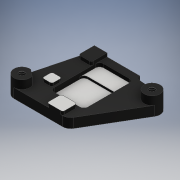
# Autodesk Inventor part: EPS_RegulatorHeatsink-A
Saved by Autodesk Inventor 2018 (Build 220112000, 112)
## iProperties
Created: 2018-09-29
Part Number: EPS_RegulatorHeatsink-A
Material: Aluminum 6061
Document SubType Name: Modeling
Designer: Bradley
Density: 2.7 g/cm^3
Appearance: Anodized - Dark Gray
Author: Bradley
Autodesk Inventor part; units mm, degrees
ref_plane "YZ Plane" through (0, 0, 0) normal (1, 0, 0) x (0, 1, 0)
ref_plane "XZ Plane" through (0, 0, 0) normal (0, 1, 0) x (-1, 0, 0)
ref_plane "XY Plane" through (0, 0, 0) normal (0, 0, 1) x (1, 0, 0)
sketch "Sketch9" plane through (0, 0, 0) normal (0, 0, 1) x (1, 0, 0)
  circle A0 centre (-9.3, -6.3) radius 2
  circle A1 centre (10.6, 6.6) radius 2
  line L0 (3.75, -3.75) -> (-3.75, -3.75) construction
  line L1 (-3.75, -3.75) -> (-3.75, 3.75) construction
  line L2 (-3.75, 3.75) -> (3.75, 3.75) construction
  line L3 (3.75, 3.75) -> (3.75, -3.75) construction
  line L4 (3.75, -3.75) -> (-3.75, 3.75) construction
  line L5 (-3.75, -3.75) -> (3.75, 3.75) construction
  line L6 (-4.95, -3.125) -> (-6.85, -3.125) construction
  line L7 (-6.85, -3.125) -> (-6.85, -1.175) construction
  line L8 (-6.85, -1.175) -> (-4.95, -1.175) construction
  line L9 (-4.95, -1.175) -> (-4.95, -3.125) construction
  line L10 (-4.95, -3.125) -> (-6.85, -1.175) construction
  line L11 (-6.85, -3.125) -> (-4.95, -1.175) construction
  line L12 (2.575, -4.925) -> (-0.575, -4.925) construction
  line L13 (-0.575, -4.925) -> (-0.575, -8.075) construction
  line L14 (-0.575, -8.075) -> (2.575, -8.075) construction
  line L15 (2.575, -8.075) -> (2.575, -4.925) construction
  line L16 (2.575, -4.925) -> (-0.575, -8.075) construction
  line L17 (-0.575, -4.925) -> (2.575, -8.075) construction
  line L18 (12.3232, 5.5848) -> (4.7232, -7.3152)
  arc A2 (3, -8.3) -> (4.7232, -7.3152) centre (3, -6.3) ccw
  line L19 (3, -8.3) -> (-9.3, -8.3)
  line L20 (-11.2363, -5.7994) -> (-7.5137, 8.5994)
  arc A3 (-7.5137, 8.5994) -> (-7.45, 9.1) centre (-9.45, 9.1) ccw
  line L21 (-7.45, 9.1) -> (-7.45, 10.1)
  line L22 (-7.45, 10.1) -> (4, 10.1)
  arc A4 (4, 10.1) -> (4.9131, 9.1038) centre (5, 10.1) ccw
  line L23 (4.9131, 9.1038) -> (10.7738, 8.5924)
  line L24 (3.25, -4.25) -> (-3.25, -4.25)
  line L25 (-4.25, -3.25) -> (-4.25, 3.25)
  line L26 (-3.25, 4.25) -> (3.25, 4.25)
  line L27 (4.25, 3.25) -> (4.25, -3.25)
  arc A5 (3.25, -4.25) -> (4.25, -3.25) centre (3.25, -3.25) ccw
  arc A6 (-4.25, -3.25) -> (-3.25, -4.25) centre (-3.25, -3.25) ccw
  arc A7 (-3.25, 4.25) -> (-4.25, 3.25) centre (-3.25, 3.25) ccw
  arc A8 (4.25, 3.25) -> (3.25, 4.25) centre (3.25, 3.25) ccw
  line L28 (1.7, 7.8) -> (-2.3, 7.8) construction
  line L29 (-2.3, 7.8) -> (-2.3, 5) construction
  line L30 (-2.3, 5) -> (1.7, 5) construction
  line L31 (1.7, 5) -> (1.7, 7.8) construction
  line L32 (1.7, 7.8) -> (-2.3, 5) construction
  line L33 (-2.3, 7.8) -> (1.7, 5) construction
  line L34 (-4.25, 3.25) -> (-4.25, 7.2)
  arc A9 (-3.25, 8.2) -> (-4.25, 7.2) centre (-3.25, 7.2) ccw
  line L35 (-3.25, 8.2) -> (3.25, 8.2)
  arc A10 (4.25, 7.2) -> (3.25, 8.2) centre (3.25, 7.2) ccw
  line L36 (4.25, 7.2) -> (4.25, 3.25)
  line L37 (-5.15, -3.4) -> (-6.65, -3.4)
  line L38 (-7.15, -2.9) -> (-7.15, -1.4)
  line L39 (-6.65, -0.9) -> (-5.15, -0.9)
  line L40 (-4.65, -1.4) -> (-4.65, -2.9)
  arc A11 (-5.15, -3.4) -> (-4.65, -2.9) centre (-5.15, -2.9) ccw
  arc A12 (-4.65, -1.4) -> (-5.15, -0.9) centre (-5.15, -1.4) ccw
  arc A13 (-6.65, -0.9) -> (-7.15, -1.4) centre (-6.65, -1.4) ccw
  arc A14 (-7.15, -2.9) -> (-6.65, -3.4) centre (-6.65, -2.9) ccw
  line L41 (2.5, -8.3) -> (-0.5, -8.3)
  line L42 (-1, -7.8) -> (-1, -5.2)
  line L43 (-0.5, -4.7) -> (2.5, -4.7)
  line L44 (3, -5.2) -> (3, -7.8)
  arc A15 (2.5, -8.3) -> (3, -7.8) centre (2.5, -7.8) ccw
  arc A16 (3, -5.2) -> (2.5, -4.7) centre (2.5, -5.2) ccw
  arc A17 (-0.5, -4.7) -> (-1, -5.2) centre (-0.5, -5.2) ccw
  arc A18 (-1, -7.8) -> (-0.5, -8.3) centre (-0.5, -7.8) ccw
  circle A19 centre (-7.6029, -4.1225) radius 1.05 construction
  line L45 (-9.3, -6.3) -> (-6.65, -2.9) construction
  line L46 (-7.4312, -5.5876) -> (-9.0655, -4.3138)
  line L47 (-4.25, 10.1) -> (-4.25, 7.2)
  line L48 (-7.45, 9.1) -> (-7.45, 6.6)
  arc A20 (-7.45, 6.6) -> (-6.95, 6.1) centre (-6.95, 6.6) ccw
  line L49 (-6.95, 6.1) -> (-4.75, 6.1)
  arc A21 (-4.75, 6.1) -> (-4.25, 6.6) centre (-4.75, 6.6) ccw
  point P0 (0, 0)
  point P1 (0, 0)
  point P2 (-5.9, -2.15)
  point P3 (1, -6.5)
  point P4 (0, 0)
  point P5 (0, -4.25)
  point P6 (0, 0)
  point P7 (-4.25, 0)
  point P8 (-0.3, 6.4)
  point P9 (1, -4.925)
  point P10 (1, -4.7)
  point P11 (-1, -6.5)
  point P12 (-0.575, -6.5)
  point P13 (-5.9, -3.4)
  point P14 (-5.9, -3.125)
  point P15 (-4.65, -2.15)
  point P16 (-4.95, -2.15)
  dimension "d71" = 4
  dimension "d72" = 19.9
  dimension "d73" = 12.9
  dimension "d74" = 9.3
  dimension "d75" = 6.3
  dimension "d76" = 7.5
  dimension "d77" = 5.9
  dimension "d78" = 2.15
  dimension "d79" = 1.9
  dimension "d80" = 1.95
  dimension "d81" = 6.5
  dimension "d82" = 1
  dimension "d83" = 3.15
  dimension "d95" = 2
  dimension "d96" = 3
  dimension "d97" = 10.1
  dimension "d103" = 1
  dimension "d104" = 8.5
  dimension "d107" = 6.4
  dimension "d108" = 2.8
  dimension "d109" = 4
  dimension "d110" = 0.3
  dimension "d111" = 1.8
  dimension "d114" = 0.5
  dimension "d115" = 0.5
  dimension "d116" = 4
  dimension "d117" = 2.5
  dimension "d118" = 2.5
  dimension "d119" = 2.1
  dimension "d120" = 1.7107
  dimension "d125" = 1
  dimension "d127" = 1
  dimension "d128" = 4
  dimension "d129" = 3.2
  dimension "d130" = 4
  constraints: 100 end point, 44 point on circle, 44 tangent, 22 centre point, 20 midpoint, 15 equal radius, 14 parallel, 14 perpendicular, 8 horizontal, 4 point on line, 3 horizontal alignment, 3 vertical, 3 vertical alignment, 2 collinear, 1 coincident, 1 line through centre
  measures "d71" diameter of A0
  measures "d72" horizontal distance of A1.centre L45.start
  measures "d73" vertical distance of L45.start A1.centre
  measures "d74" horizontal distance of L45.start point (0, 0)
  measures "d75" vertical distance of L45.start point (0, 0)
  measures "d76" distance of L1.end L2.end
  measures "d77" horizontal distance of point (-5.9, -2.15) point (0, 0)
  measures "d78" vertical distance of point (-5.9, -2.15) point (0, 0)
  measures "d79" distance of L7.end L8.end
  measures "d80" distance of L6.end L7.end
  measures "d81" vertical distance of point (1, -6.5) point (0, 0)
  measures "d82" horizontal distance of point (1, -6.5) point (0, 0)
  measures "d83" distance of L12.start L12.end
  measures "d95" radius of A2
  measures "d96" horizontal distance of point (0, 0) A2.centre
  measures "d97" distance from line of point (0, 0) L22
  measures "d103" radius of A5
  measures "d104" distance between parallel lines of L25 L27
  measures "d107" vertical distance of point (-0.3, 6.4) point (0, 0)
  measures "d108" distance of L30.end L28.start
  measures "d109" distance of L29.end L30.end
  measures "d110" horizontal distance of point (0, 0) point (-0.3, 6.4)
  measures "d111" distance from line of point (-0.3, 6.4) L35
  measures "d114" radius of A11
  measures "d115" radius of A15
  measures "d116" distance between parallel lines of L42 L44
  measures "d117" distance between parallel lines of L39 L37
  measures "d118" distance between parallel lines of L40 L38
  measures "d119" diameter of A19
  measures "d120" distance from line of L46 L45.start
  measures "d125" distance of L21.start L21.end
  measures "d127" radius of A4
  measures "d128" horizontal distance of L22.end point (0, 0)
  measures "d129" distance between parallel lines of L21 L34
  measures "d130" distance between parallel lines of L22 L49
extrude "Extrusion7" add sketch "Sketch9" along normal blind 3.5 and the other way blind 1 contours A0 L46 | A1 picked at (-9.5, -5.1238)
sketch "Sketch10" plane through (10.6, 6.6, 3.5) normal (0, 0, 1) x (1, 0, 0)
  arc A0 (-19.6655, -10.9138) -> (-18.0312, -12.1876) centre (-19.9, -12.9) ccw projected
  circle A1 centre (0, 0) radius 2 projected
  line L0 (-18.0312, -12.1876) -> (-19.6655, -10.9138) projected
  point P0 (-10.6, -6.6)
hole "Hole3" at (10.6, 6.6, 3.5) at (-9.3, -6.3, 3.5) direction (0, 0, -1) diameter 1.567 end through all thread size "M2x0.4" class "6H" standard "ANSI Metric M Profile"
extrude "Extrusion8" add sketch "Sketch9" against normal up to surface (1 mm away) contours A0 L20 A3 L48 A20 L49 A21 L34 L25 A6 L24 A5 L27 L36 A10 L35 A9 L47 L22 A4 L23 A1 L18 A2 L19 A15 L44 A16 L43 A17 L42 A18 | L46 A0 | A18 L42 A17 L43 A16 L44 A15 L19 | L21 L22 L47 L34 A21 L49 A20 L48 | A9 L35 A10 L36 A8 L26 A7 L34 | A7 L26 A8 L27 A5 L24 A6 L25 | L37 A14 L38 A13 L39 A12 L40 A11 picked at (-8.1343, -4.9223)
extrude "Extrusion9" add sketch "Sketch9" along normal blind 0.5 contours A0 L20 A3 L48 A20 L49 A21 L34 L25 A6 L24 A5 L27 L36 A10 L35 A9 L47 L22 A4 L23 A1 L18 A2 L19 A15 L44 A16 L43 A17 L42 A18 | L46 A0 | A18 L42 A17 L43 A16 L44 A15 L19 | L21 L22 L47 L34 A21 L49 A20 L48 | A9 L35 A10 L36 A8 L26 A7 L34 | L37 A14 L38 A13 L39 A12 L40 A11 picked at (-8.1343, -4.9223)
extrude "Extrusion10" add sketch "Sketch9" along normal blind 1.4 contours A0 L20 A3 L48 A20 L49 A21 L34 L25 A6 L24 A5 L27 L36 A10 L35 A9 L47 L22 A4 L23 A1 L18 A2 L19 A15 L44 A16 L43 A17 L42 A18 | L46 A0 | A18 L42 A17 L43 A16 L44 A15 L19 | L21 L22 L47 L34 A21 L49 A20 L48 | L37 A14 L38 A13 L39 A12 L40 A11 picked at (-8.1343, -4.9223)
extrude "Extrusion11" add sketch "Sketch9" along normal blind 2.27 contours A18 L42 A17 L43 A16 L44 A15 L19
extrude "Extrusion12" add sketch "Sketch9" along normal blind 2.15 contours L37 A14 L38 A13 L39 A12 L40 A11
extrude "Extrusion13" add sketch "Sketch9" along normal blind 2.3 contours L21 L22 L47 L34 A21 L49 A20 L48
sketch "Sketch11" plane through (-7.45, 10.1, -1) normal (0, 1, 0) x (1, 0, 0)
  line L0 (0, 0) -> (0, -3.3) projected
  line L1 (3.2, -3.3) -> (0, -3.3) projected
  line L2 (3.2, -2.4) -> (3.2, -3.3) projected
  line L3 (11.45, -2.4) -> (3.2, -2.4) projected
  line L4 (11.45, 0) -> (11.45, -2.4) projected
  line L5 (0, 0) -> (11.45, 0) projected
  line L6 (0, 0) -> (11.45, 0) construction
  line L7 (0, 0) -> (3.2, -3.3) construction
  point P0 (7.45, -1)
  point P1 (1.6, -1.65)
  constraints: 2 end point, 1 midpoint
hole "Hole4" at (-5.85, 10.1, 0.65) direction (0, -1, 0) diameter 1.221 depth 3 tip angle 118 thread size "M1.6x0.35" class "6H" standard "ANSI Metric M Profile"
equation "\"SilPad\" = 0.35"
body "Solid2"
